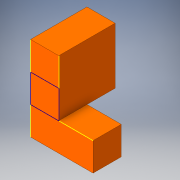
# Autodesk Inventor part: IED7_Sun_PuzzleCubeOrange
Saved by Autodesk Inventor 2016 (Build 200138000, 138)
## iProperties
Created: 2017-09-28
Part Number: IED7_Sun_PuzzleCubeOrange
Material: Generic
Document SubType Name: Sheet Metal
Designer: sun01147
Density: 1 g/cm^3
Sheet Metal Rule: Default
Appearance: Default
Author: sun01147
Autodesk Inventor part; units mm, degrees
ref_plane "YZ Plane" through (0, 0, 0) normal (1, 0, 0) x (0, 1, 0)
ref_plane "XZ Plane" through (0, 0, 0) normal (0, 1, 0) x (-1, 0, 0)
ref_plane "XY Plane" through (0, 0, 0) normal (0, 0, 1) x (1, 0, 0)
sketch "Sketch1" plane through (0, 0, 0) normal (0, 0, 1) x (1, 0, 0)
  line L0 (0, 19.05) -> (0, 0)
  line L1 (0, 19.05) -> (42.2604, 19.05)
  line L2 (42.2604, 19.05) -> (42.2604, 0)
  line L3 (42.2604, 0) -> (0, 0)
  line L4 (0, 19.05) -> (0, 57.15)
  line L5 (0, 57.15) -> (19.05, 57.15)
  line L6 (19.05, 57.15) -> (19.05, 19.05)
  line L7 (0, 38.1) -> (19.05, 38.1)
  dimension "d0" = 19.05
  dimension "d1" = 19.05
  dimension "d2" = 38.1
  constraints: 16 end point, 4 perpendicular, 2 midpoint, 2 vertical, 1 horizontal, 1 point on line
  measures "d0" distance of L0.start L0.end
  measures "d1" distance of L4.end L5.end
  measures "d2" distance of L0.start L4.end
extrude "Extrusion1" add sketch "Sketch1" against normal blind 19.05
sketch "straight 3 cube" plane through (0, 0, 0) normal (0, 0, 1) x (1, 0, 0)
  line L0 (19.05, 19.05) -> (42.2604, 19.05) projected
  line L1 (19.05, 19.05) -> (0, 19.05)
  line L2 (0, 0) -> (0, 57.15) projected
  line L3 (19.05, 19.05) -> (19.05, 38.1)
  line L4 (19.05, 57.15) -> (19.05, 19.05) projected
  line L5 (19.05, 38.1) -> (0, 38.1)
  line L6 (19.05, 19.05) -> (0, 19.05)
  line L7 (19.05, 19.05) -> (0, 19.05)
  line L8 (19.05, 19.05) -> (19.05, 38.1)
  line L9 (0, 38.1) -> (19.05, 38.1)
  line L10 (19.05, 38.1) -> (0, 38.1)
  line L11 (0, 38.1) -> (0, 19.05)
  line L12 (0, 19.05) -> (19.05, 19.05)
  line L13 (19.05, 19.05) -> (19.05, 38.1)
  line L14 (19.05, 19.05) -> (0, 19.05)
  constraints: 24 end point, 5 collinear, 2 horizontal, 2 parallel, 2 perpendicular, 2 point on line, 1 midpoint
sketch "Sketch3" plane through (0, 0, -19.05) normal (0, 0, -1) x (-1, 0, 0)
  line L0 (-19.05, 19.05) -> (-42.2604, 19.05) projected
  line L1 (-19.05, 19.05) -> (0, 19.05)
  line L2 (0, 0) -> (0, 57.15) projected
  line L3 (0, 19.05) -> (0, 57.15)
  line L4 (0, 57.15) -> (-19.05, 57.15) projected
  line L5 (0, 57.15) -> (-19.05, 57.15)
  line L6 (-19.05, 57.15) -> (-19.05, 19.05) projected
  line L7 (-19.05, 57.15) -> (-19.05, 19.05)
  constraints: 8 end point, 4 collinear, 1 point on line
extrude "Extrusion2" add sketch "Sketch3" along normal blind 19.05
equation "\"d1\" = cube"
equation "\"d2\" = 2 * cube"
equation "\"d3\" = cube"
equation "\"d5\" = cube"
equation "\"BendRadius\" = Thickness"
equation "\"BendReliefWidth\" = Thickness"
equation "\"BendReliefDepth\" = 0.5 * Thickness"
equation "\"CornerReliefSize\" = 4 * Thickness"
equation "\"MinimumRemnant\" = 2 * Thickness"
equation "\"TransitionRadius\" = BendRadius"
equation "\"JacobiRadiusSize\" = BendRadius"
equation "\"GapSize\" = Thickness"
equation "\"cube\" = 19.05"
equation "\"Thickness\" = 3.048"
body "Solid1"
